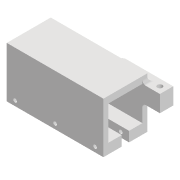
# Autodesk Inventor part: Motor_mount
Saved by Autodesk Inventor 2022 (Build 260153000, 153)
## iProperties
Created: 2022-05-04
Part Number: Motor_mount
Material: Generic
Document SubType Name: Modeling
Designer: dell
Density: 1 g/cm^3
Appearance: Default
Author: dell
Autodesk Inventor part; units mm, degrees
ref_plane "YZ Plane" through (0, 0, 0) normal (1, 0, 0) x (0, 1, 0)
ref_plane "XZ Plane" through (0, 0, 0) normal (0, 1, 0) x (-1, 0, 0)
ref_plane "XY Plane" through (0, 0, 0) normal (0, 0, 1) x (1, 0, 0)
sketch "Sketch2" plane through (0, 0, 0) normal (1, 0, 0) x (0, 1, 0)
  line L0 (26.9971, -5.0019) -> (6.5971, -5.0019)
  line L1 (6.5971, -5.0019) -> (6.5971, -25.4019)
  line L2 (6.5971, -25.4019) -> (26.9971, -25.4019)
  line L3 (26.9971, -25.4019) -> (26.9971, -5.0019)
  line L4 (30.9971, -2.0019) -> (0.5971, -2.0019)
  line L5 (30.9971, -28.4019) -> (30.9971, -2.0019)
  line L6 (0.5971, -2.0019) -> (0.5971, -28.4019)
  line L7 (30.9971, -28.4019) -> (0.5971, -28.4019)
  line L8 (6.5971, -13.0019) -> (0.5971, -13.0019)
  line L9 (0.5971, -13.0019) -> (0.5971, -17.4019)
  line L10 (0.5971, -17.4019) -> (6.5971, -17.4019)
  line L11 (6.5971, -17.4019) -> (6.5971, -13.0019)
  point P0 (0, 0)
  point P1 (0.5971, -13.0019)
  dimension "d5" = 20.4
  dimension "d6" = 20.4
  dimension "d8" = 6
  dimension "d22" = 4
  dimension "d23" = 3
  dimension "d24" = 3
  dimension "d27" = 8
  dimension "d28" = 8
  constraints: 24 end point, 4 parallel, 3 horizontal, 2 perpendicular, 2 point on line, 1 vertical
  measures "d5" distance of L0.start L0.end
  measures "d6" distance of L0.end L1.end
  measures "d8" distance between parallel lines of L1 L6
  measures "d22" distance between parallel lines of L5 L3
  measures "d23" distance between parallel lines of L2 L7
  measures "d24" distance between parallel lines of L4 L0
  measures "d27" distance from line of L0.end L8
  measures "d28" distance from line of L1.end L10
extrude "Extrusion1" add sketch "Sketch2" along normal blind 54.8 contours L0 L1 L8 L6 L4 L5 L7 L10 L2 L3
sketch "Sketch4" plane through (0, 0.5971, -28.4019) normal (0, 0, -1) x (-1, 0, 0)
  line L0 (0, 6) -> (0, 26.4) projected
  line L1 (0, 26.4) -> (-54.8, 26.4) projected
  line L2 (-54.8, 6) -> (-54.8, 26.4) projected
  line L3 (0, 6) -> (-54.8, 6) projected
  line L4 (0, 26.4) -> (-54.8, 26.4) projected
  line L5 (-54.8, 26.4) -> (-83.55, 26.4)
  line L6 (-83.55, 26.4) -> (-83.55, 16.4)
  line L7 (-83.55, 16.4) -> (-54.8, 16.4)
  line L8 (-54.8, 16.4) -> (-54.8, 26.4)
  line L9 (-43.55, 26.4) -> (-43.55, 16.4) construction
  point P0 (0, -0.5971)
  dimension "d29" = 10
  dimension "d30" = 11.25
  dimension "d31" = 40
  dimension "d32" = 0
  constraints: 10 end point, 3 point on line, 2 parallel, 2 perpendicular, 1 horizontal
  measures "d29" distance between parallel lines of L1 L7
  measures "d30" distance between parallel lines of L2 L9
  measures "d31" distance between parallel lines of L6 L9
  measures "d32" distance between parallel lines of L2 L8
extrude "Extrusion3" add sketch "Sketch4" along normal blind 5 and the other way blind 3 contours L2 L7 L6 L5
sketch "Sketch10" plane through (54.8, 26.9971, -33.4019) normal (0, 1, 0) x (1, 0, 0)
  line L0 (28.75, -8) -> (0, -8) projected
  line L1 (28.75, -8) -> (28.75, 0) projected
  line L2 (0, 0) -> (28.75, 0) projected
  line L3 (0, 0) -> (0, -5) projected
  circle A0 centre (24.75, -4) radius 1.5
  line L4 (0, -8) -> (0, -5) projected
  point P0 (-54.8, -33.4019)
  dimension "d55" = 3
  dimension "d56" = 4
  dimension "d57" = 4
  constraints: 1 centre point
  measures "d55" diameter of A0
  measures "d56" distance from line of L1 A0.centre
  measures "d57" distance from line of L0 A0.centre
extrude "Extrusion8" cut sketch "Sketch10" against normal blind 10 contours A0
sketch "Sketch11" plane through (54.8, 0, 0) normal (1, 0, 0) x (0, 0, -1)
  line L0 (25.4019, 26.9971) -> (28.4019, 26.9971) projected
  line L1 (28.4019, 26.9971) -> (28.4019, 30.9971) projected
  line L2 (28.4019, 30.9971) -> (2.0019, 30.9971) projected
  line L3 (2.0019, 30.9971) -> (2.0019, 0.5971) projected
  line L4 (2.0019, 0.5971) -> (13.0019, 0.5971) projected
  line L5 (13.0019, 0.5971) -> (13.0019, 6.5971) projected
  line L6 (13.0019, 6.5971) -> (5.0019, 6.5971) projected
  line L7 (5.0019, 6.5971) -> (5.0019, 26.9971) projected
  line L8 (5.0019, 26.9971) -> (25.4019, 26.9971) projected
  line L9 (28.4019, 16.9971) -> (25.4019, 16.9971) projected
  line L10 (25.4019, 16.9971) -> (25.4019, 6.5971) projected
  line L11 (25.4019, 6.5971) -> (17.4019, 6.5971) projected
  line L12 (17.4019, 6.5971) -> (17.4019, 0.5971) projected
  line L13 (17.4019, 0.5971) -> (28.4019, 0.5971) projected
  line L14 (28.4019, 0.5971) -> (28.4019, 16.9971) projected
  point P0 (0, 0)
extrude "Extrusion9" add sketch "Sketch11" along normal blind 15
fillet "Fillet3" radius 2 6 edges at (62.3, 26.9971, -28.4019) (54.8, 21.9971, -28.4019) (62.3, 16.9971, -28.4019) (69.8, 26.9971, -26.9019) (69.8, 16.9971, -26.9019) (54.8, 21.9971, -33.4019)
sketch "Sketch12" plane through (0, 0.5971, -28.4019) normal (0, 0, -1) x (-1, 0, 0)
  line L0 (0, 0) -> (0, 6) projected
  line L1 (0, 6) -> (-69.8, 6) projected
  line L2 (-69.8, 0) -> (-69.8, 6) projected
  line L3 (0, 0) -> (-69.8, 0) projected
  circle A0 centre (-64.8, 3) radius 1.1
  circle A1 centre (-40.8, 3) radius 1.1
  circle A2 centre (-5, 3) radius 1.1
  point P0 (0, -0.5971)
  dimension "d64" = 2.2
  dimension "d65" = 5
  dimension "d66" = 3
  dimension "d67" = 2.2
  dimension "d68" = 2.2
  dimension "d69" = 5
  dimension "d70" = 3
  dimension "d71" = 29
  dimension "d72" = 3
  constraints: 3 centre point
  measures "d64" diameter of A0
  measures "d65" distance from line of L2 A0.centre
  measures "d66" distance from line of L3 A0.centre
  measures "d67" diameter of A1
  measures "d68" diameter of A2
  measures "d69" distance from line of L0 A2.centre
  measures "d70" distance from line of L3 A2.centre
  measures "d71" distance from line of L2 A1.centre
  measures "d72" distance from line of L3 A1.centre
extrude "Extrusion10" cut sketch "Sketch12" against normal blind 100 contours A0 | A1 | A2
sketch "Sketch13" plane through (0, 30.9971, -2.0019) normal (0, 1, 0) x (1, 0, 0)
  line L0 (0, 0) -> (69.8, 0) projected
  line L1 (0, 26.4) -> (69.8, 26.4) projected
  line L2 (54.8, 0) -> (50.8, 0)
  line L3 (50.8, 0) -> (50.8, 26.4)
  line L4 (50.8, 26.4) -> (54.8, 26.4)
  line L5 (54.8, 26.4) -> (54.8, 0)
  line L6 (4, 0) -> (0, 0)
  line L7 (0, 0) -> (0, 26.4)
  line L8 (0, 26.4) -> (4, 26.4)
  line L9 (4, 26.4) -> (4, 0)
  line L10 (0, 26.4) -> (0, 0) projected
  point P0 (0, -2.0019)
  point P1 (4, 0)
  point P2 (50.8, 0)
  dimension "d75" = 4
  dimension "d76" = 4
  dimension "d77" = 46.8
  constraints: 16 end point, 4 parallel, 4 point on line, 2 horizontal, 2 perpendicular, 1 collinear
  measures "d75" distance between parallel lines of L5 L3
  measures "d76" distance between parallel lines of L9 L7
  measures "d77" distance between parallel lines of L3 L9
extrude "Extrusion11" add sketch "Sketch13" along normal blind 27 contours L7 L1 L9 L0 | L3 L1 L5 L0
sketch "Sketch14" plane through (54.8, 30.9971, -2.0019) normal (1, 0, 0) x (0, 0, -1)
  circle A0 centre (6.25, 11) radius 1.3
  line L0 (26.4, 0) -> (0, 0) projected
  circle A1 centre (6.25, 23) radius 1.3
  line L1 (0, 0) -> (0, 27) projected
  circle A2 centre (20.15, 23) radius 1.3
  circle A3 centre (20.15, 11) radius 1.3
  line L2 (26.4, 0) -> (26.4, 27) projected
  point P0 (-2.0019, -30.9971)
  dimension "d80" = 2.6
  dimension "d81" = 11
  dimension "d82" = 2.6
  dimension "d83" = 23
  dimension "d84" = 6.25
  dimension "d85" = 6.25
  dimension "d86" = 2.6
  dimension "d87" = 2.6
  dimension "d88" = 11
  dimension "d89" = 23
  dimension "d90" = 6.25
  dimension "d91" = 6.25
  constraints: 4 centre point
  measures "d80" diameter of A0
  measures "d81" distance from line of L0 A0.centre
  measures "d82" diameter of A1
  measures "d83" distance from line of L0 A1.centre
  measures "d84" distance from line of L1 A1.centre
  measures "d85" distance from line of L1 A0.centre
  measures "d86" diameter of A2
  measures "d87" diameter of A3
  measures "d88" distance from line of L0 A3.centre
  measures "d89" distance from line of L0 A2.centre
  measures "d90" distance from line of L2 A3.centre
  measures "d91" distance from line of L2 A2.centre
extrude "Extrusion12" cut sketch "Sketch14" against normal blind 100
fillet "Fillet4" radius 2 1 edges at (54.8, 30.9971, -15.2019)
body "Solid1"
